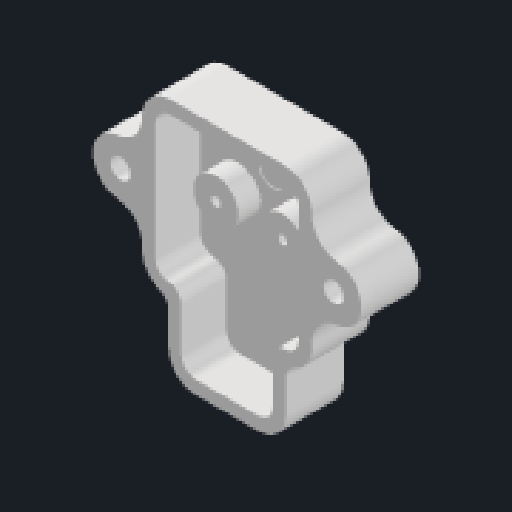
# Autodesk Inventor part: pressure_housing
Saved by Autodesk Inventor 2024 (Build 280153000, 153)
## iProperties
Created: 2025-03-06
Part Number: pressure_housing
Material: Generic
Document SubType Name: Modeling
Designer: colel
Density: 1 g/cm^3
Appearance: Default
Author: colel
Autodesk Inventor part; units mm, degrees
ref_plane "YZ Plane" through (0, 0, 0) normal (1, 0, 0) x (0, 1, 0)
ref_plane "XZ Plane" through (0, 0, 0) normal (0, 1, 0) x (-1, 0, 0)
ref_plane "XY Plane" through (0, 0, 0) normal (0, 0, 1) x (1, 0, 0)
sketch "Sketch1" plane through (0, 0, 0) normal (0, 0, 1) x (1, 0, 0)
  circle A0 centre (0, 0) radius 3
  circle A1 centre (7.5, -7) radius 1
  circle A2 centre (-7.5, -7) radius 1
  line L0 (-7.5, -7) -> (7.5, -7) construction
  line L1 (-19.05, 12.7) -> (19.05, 12.7)
  line L2 (19.05, 12.7) -> (19.05, -26.05)
  line L3 (19.05, -26.05) -> (-19.05, -26.05)
  line L4 (-19.05, -26.05) -> (-19.05, 12.7)
  circle A3 centre (-7.5, -7) radius 5
  circle A4 centre (7.5, -7) radius 5
  line L5 (16.05, 9.7) -> (-16.05, 9.7)
  line L6 (-16.05, 9.7) -> (-16.05, -23.05)
  line L7 (-16.05, -23.05) -> (16.05, -23.05)
  line L8 (16.05, -23.05) -> (16.05, 9.7)
  point P0 (0, -7)
  point P1 (0, 12.7)
  point P2 (16.05, -10.1819)
  point P3 (16.05, -2.5181)
  point P4 (-16.05, -2.5181)
  point P5 (-16.05, -10.1819)
  dimension "d0" = 7
  dimension "d1" = 15
  dimension "d2" = 6
  dimension "d3" = 2
  dimension "d4" = 38.1
  dimension "d5" = 12.7
  dimension "d6" = 19.05
  dimension "d7" = 4
  dimension "d8" = 3
  constraints: 18 end point, 5 centre point, 4 parallel, 3 coincident, 2 equal radius, 2 horizontal, 2 midpoint, 2 perpendicular, 2 vertical alignment, 1 horizontal alignment, 3 other
  measures "d0" distance from line of point (0, 0) L0
  measures "d1" distance of L0.start L0.end
  measures "d2" diameter of A0
  measures "d3" diameter of A2
  measures "d4" distance of L1.start L1.end
  measures "d5" distance from line of L1 point (0, 0)
  measures "d6" distance between parallel lines of L3 L0
  measures "d7" radial gap between concentric circles of A3 A2
  measures "d8" distance between parallel lines of L1 L5
extrude "Extrusion1" add sketch "Sketch1" against normal blind 3 contours A0 | A1 | A2 | L1 L2 L3 L4 | A3 | A4 | L8 L7 L6 L5
extrude "Extrusion2" add sketch "Sketch1" along normal blind 10 contours L1 L2 L3 L4
extrude "Extrusion3" add sketch "Sketch1" along normal blind 5 contours A3 | A4
extrude "Extrusion4" cut sketch "Sketch1" against normal blind 0.25 contours A0
fillet "Fillet1" radius 3.175 4 edges at (16.05, 9.7, 5) (16.05, -23.05, 5) (-16.05, -23.05, 5) (-16.05, 9.7, 5)
fillet "Fillet2" radius 6.175 4 edges at (-19.05, 12.7, 3.5) (-19.05, -26.05, 3.5) (19.05, -26.05, 3.5) (19.05, 12.7, 3.5)
sketch "Sketch2" plane through (0, 0, -3) normal (0, 0, -1) x (-1, 0, 0)
  line L0 (-7.075, -32.6439) -> (5.625, -32.6439) projected
  arc A0 (5.625, -38.9939) -> (5.625, -32.6439) centre (5.625, -35.8189) ccw projected
  line L1 (5.625, -38.9939) -> (-7.075, -38.9939) projected
  arc A1 (-7.075, -32.6439) -> (-7.075, -38.9939) centre (-7.075, -35.8189) ccw projected
  circle A2 centre (-22.0588, 28.4811) radius 1.5 projected
  circle A3 centre (32.925, -38.8189) radius 1.5 projected
  circle A4 centre (32.925, 7.1488) radius 1.5 projected
  circle A5 centre (-34.375, 7.1488) radius 1.5 projected
  circle A6 centre (-34.375, -38.8189) radius 1.5 projected
  circle A7 centre (20.6088, 28.4811) radius 1.5 projected
  arc A8 (39.275, 7.1488) -> (38.4243, 10.3238) centre (32.925, 7.1488) ccw projected
  line L2 (26.1081, 31.6561) -> (38.4243, 10.3238) projected
  arc A9 (26.1081, 31.6561) -> (20.6088, 34.8311) centre (20.6088, 28.4811) ccw projected
  line L3 (20.6088, 34.8311) -> (-22.0588, 34.8311) projected
  arc A10 (-22.0588, 34.8311) -> (-27.5581, 31.6561) centre (-22.0588, 28.4811) ccw projected
  line L4 (-39.8743, 10.3238) -> (-27.5581, 31.6561) projected
  arc A11 (-39.8743, 10.3238) -> (-40.725, 7.1488) centre (-34.375, 7.1488) ccw projected
  line L5 (-40.725, -38.8189) -> (-40.725, 7.1488) projected
  arc A12 (-40.725, -38.8189) -> (-34.375, -45.1689) centre (-34.375, -38.8189) ccw projected
  line L6 (32.925, -45.1689) -> (-34.375, -45.1689) projected
  arc A13 (32.925, -45.1689) -> (39.275, -38.8189) centre (32.925, -38.8189) ccw projected
  line L7 (39.275, 7.1488) -> (39.275, -38.8189) projected
  circle A14 centre (0, 0) radius 3 projected
  arc A15 (-12.875, 12.7) -> (-19.05, 6.525) centre (-12.875, 6.525) ccw projected
  line L8 (-19.05, 6.525) -> (-19.05, -19.875) projected
  arc A16 (-19.05, -19.875) -> (-12.875, -26.05) centre (-12.875, -19.875) ccw projected
  line L9 (-12.875, -26.05) -> (12.875, -26.05) projected
  arc A17 (12.875, -26.05) -> (19.05, -19.875) centre (12.875, -19.875) ccw projected
  line L10 (19.05, -19.875) -> (19.05, 6.525) projected
  arc A18 (19.05, 6.525) -> (12.875, 12.7) centre (12.875, 6.525) ccw projected
  line L11 (12.875, 12.7) -> (-12.875, 12.7) projected
  line L12 (-13.25, -45.1689) -> (-13.25, -26.0386)
  line L13 (-12.875, -26.05) -> (12.875, -26.05) projected
  line L14 (13.25, -45.1689) -> (13.25, -26.0386)
  line L15 (-13.25, -35.8189) -> (13.25, -35.8189) construction
  line L16 (-7.075, -41.9939) -> (7.075, -41.9939)
  arc A19 (5.625, -41.9939) -> (5.625, -29.6439) centre (5.625, -35.8189) ccw construction
  line L17 (7.075, -29.6439) -> (-7.075, -29.6439)
  arc A20 (-7.075, -29.6439) -> (-7.075, -41.9939) centre (-7.075, -35.8189) ccw
  arc A21 (6.35, -29.6866) -> (6.35, -41.9512) centre (7.075, -35.8189) ccw construction
  arc A22 (7.075, -41.9939) -> (7.075, -29.6439) centre (7.075, -35.8189) ccw
  line L18 (12.875, -26.05) -> (-12.875, -26.05) projected
  line L19 (-10.25, -26.05) -> (-10.25, -30.5227)
  line L20 (10.25, -26.05) -> (10.25, -30.5227)
  line L21 (-10.25, -30.5227) -> (-10.25, -35.8189)
  line L22 (10.25, -30.5227) -> (10.25, -35.8189)
  circle A23 centre (7.075, -35.8189) radius 3.175
  line L23 (5.625, -38.9939) -> (7.075, -38.9939)
  circle A24 centre (23.9875, -6.35) radius 1.5 projected
  circle A25 centre (-23.9875, -6.35) radius 1.5 projected
  point P0 (0, 0)
  point P1 (0, -35.8189)
  point P2 (0, -26.05)
  point P3 (-13.25, -35.8189)
  dimension "d19" = 6.175
  dimension "d20" = 3
  dimension "d21" = 3
  constraints: 20 end point, 17 point on circle, 11 point on line, 5 centre point, 3 perpendicular, 3 tangent, 2 midpoint, 2 vertical, 1 coincident, 1 parallel, 1 vertical alignment
  measures "d19" distance from line of L12 A1.centre
  measures "d20" distance between parallel lines of L19 L12
  measures "d21" distance between parallel lines of L14 L20
extrude "Extrusion5" add sketch "Sketch2" against normal up to surface (13 mm away) contours A1 L1 L23 A23 L22 A22 L16 A20 L21 | A20 L12 A16 L9 L19 | L20 L9 A17 L14 A22
sketch "Sketch3" plane through (0, 0, -3) normal (0, 0, -1) x (-1, 0, 0)
  line L0 (-10.25, -26.05) -> (10.25, -26.05) projected
  line L1 (10.25, -26.05) -> (10.25, -35.8189) projected
  arc A0 (7.075, -38.9939) -> (10.25, -35.8189) centre (7.075, -35.8189) ccw projected
  line L2 (7.075, -38.9939) -> (-7.075, -38.9939) projected
  arc A1 (-10.25, -35.8189) -> (-7.075, -38.9939) centre (-7.075, -35.8189) ccw projected
  line L3 (-10.25, -35.8189) -> (-10.25, -26.05) projected
  line L4 (-13.25, -26.0386) -> (-13.25, -35.8189) projected
  arc A2 (-13.25, -35.8189) -> (-7.075, -41.9939) centre (-7.075, -35.8189) ccw projected
  line L5 (-7.075, -41.9939) -> (7.075, -41.9939) projected
  arc A3 (7.075, -41.9939) -> (13.25, -35.8189) centre (7.075, -35.8189) ccw projected
  line L6 (13.25, -35.8189) -> (13.25, -26.0386) projected
  arc A4 (13.25, -26.0386) -> (19.05, -19.875) centre (12.875, -19.875) ccw projected
  line L7 (19.05, -19.875) -> (19.05, 6.525) projected
  arc A5 (19.05, 6.525) -> (12.875, 12.7) centre (12.875, 6.525) ccw projected
  line L8 (12.875, 12.7) -> (-12.875, 12.7) projected
  arc A6 (-12.875, 12.7) -> (-19.05, 6.525) centre (-12.875, 6.525) ccw projected
  line L9 (-19.05, 6.525) -> (-19.05, -19.875) projected
  arc A7 (-19.05, -19.875) -> (-13.25, -26.0386) centre (-12.875, -19.875) ccw projected
  point P0 (0, 0)
extrude "Extrusion6" add sketch "Sketch3" against normal blind 3 contours L0 L1 A0 L2 A1 L3
sketch "Sketch4" plane through (0, 0, 10) normal (0, 0, 1) x (1, 0, 0)
  arc A0 (13.25, -26.0386) -> (19.05, -19.875) centre (12.875, -19.875) ccw projected
  line L0 (19.05, -19.875) -> (19.05, 6.525) projected
  arc A1 (19.05, 6.525) -> (12.875, 12.7) centre (12.875, 6.525) ccw projected
  line L1 (12.875, 12.7) -> (-12.875, 12.7) projected
  arc A2 (-12.875, 12.7) -> (-19.05, 6.525) centre (-12.875, 6.525) ccw projected
  line L2 (-19.05, 6.525) -> (-19.05, -19.875) projected
  arc A3 (-19.05, -19.875) -> (-13.25, -26.0386) centre (-12.875, -19.875) ccw projected
  line L3 (-13.25, -35.8189) -> (-13.25, -26.0386) projected
  arc A4 (-13.25, -35.8189) -> (-7.075, -41.9939) centre (-7.075, -35.8189) ccw projected
  line L4 (7.075, -41.9939) -> (-7.075, -41.9939) projected
  arc A5 (7.075, -41.9939) -> (13.25, -35.8189) centre (7.075, -35.8189) ccw projected
  line L5 (13.25, -26.0386) -> (13.25, -35.8189) projected
  line L6 (10.25, -35.8189) -> (10.25, -26.05) projected
  arc A6 (7.075, -38.9939) -> (10.25, -35.8189) centre (7.075, -35.8189) ccw projected
  line L7 (-7.075, -38.9939) -> (7.075, -38.9939) projected
  arc A7 (-10.25, -35.8189) -> (-7.075, -38.9939) centre (-7.075, -35.8189) ccw projected
  line L8 (-10.25, -26.05) -> (-10.25, -35.8189) projected
  line L9 (-10.25, -26.05) -> (10.25, -26.05) projected
  line L10 (-12.875, 9.7) -> (12.875, 9.7) projected
  arc A8 (16.05, 6.525) -> (12.875, 9.7) centre (12.875, 6.525) ccw projected
  line L11 (16.05, 6.525) -> (16.05, -19.875) projected
  arc A9 (12.875, -23.05) -> (16.05, -19.875) centre (12.875, -19.875) ccw projected
  line L12 (12.875, -23.05) -> (-12.875, -23.05) projected
  arc A10 (-16.05, -19.875) -> (-12.875, -23.05) centre (-12.875, -19.875) ccw projected
  line L13 (-16.05, -19.875) -> (-16.05, 6.525) projected
  arc A11 (-12.875, 9.7) -> (-16.05, 6.525) centre (-12.875, 6.525) ccw projected
  line L14 (-10.25, -26.05) -> (-10.25, -23.05)
  line L15 (10.25, -26.05) -> (10.25, -23.05)
  point P0 (0, 0)
  constraints: 4 end point, 2 point on line, 2 vertical
extrude "Extrusion7" cut sketch "Sketch4" against normal up to surface (10 mm away) contours L9 L14 L12 L15
fillet "Fillet3" radius 3 4 edges at (-10.25, -23.05, 5) (-13.25, -26.0386, 3.5) (13.25, -26.0386, 3.5) (10.25, -23.05, 5)
sketch "Sketch5" plane through (0, 0, -3) normal (0, 0, -1) x (-1, 0, 0)
  arc A0 (-10.25, -26.0386) -> (-13.0678, -23.0441) centre (-13.25, -26.0386) ccw projected
  line L0 (-10.25, -35.8189) -> (-10.25, -26.0386) projected
  arc A1 (-10.25, -35.8189) -> (-7.075, -38.9939) centre (-7.075, -35.8189) ccw projected
  line L1 (7.075, -38.9939) -> (-7.075, -38.9939) projected
  arc A2 (7.075, -38.9939) -> (10.25, -35.8189) centre (7.075, -35.8189) ccw projected
  line L2 (10.25, -35.8189) -> (10.25, -26.0386) projected
  arc A3 (13.0678, -23.0441) -> (10.25, -26.0386) centre (13.25, -26.0386) ccw projected
  arc A4 (13.0678, -23.0441) -> (16.05, -19.875) centre (12.875, -19.875) ccw projected
  line L3 (16.05, -19.875) -> (16.05, 6.525) projected
  arc A5 (16.05, 6.525) -> (12.875, 9.7) centre (12.875, 6.525) ccw projected
  line L4 (12.875, 9.7) -> (-12.875, 9.7) projected
  arc A6 (-12.875, 9.7) -> (-16.05, 6.525) centre (-12.875, 6.525) ccw projected
  line L5 (-16.05, 6.525) -> (-16.05, -19.875) projected
  arc A7 (-16.05, -19.875) -> (-13.0678, -23.0441) centre (-12.875, -19.875) ccw projected
  arc A8 (-19.05, -19.875) -> (-15.1465, -25.617) centre (-12.875, -19.875) ccw projected
  line L6 (-19.05, -19.875) -> (-19.05, 6.525) projected
  arc A9 (-12.875, 12.7) -> (-19.05, 6.525) centre (-12.875, 6.525) ccw projected
  line L7 (-12.875, 12.7) -> (12.875, 12.7) projected
  arc A10 (19.05, 6.525) -> (12.875, 12.7) centre (12.875, 6.525) ccw projected
  line L8 (19.05, 6.525) -> (19.05, -19.875) projected
  arc A11 (15.1465, -25.617) -> (19.05, -19.875) centre (12.875, -19.875) ccw projected
  arc A12 (15.1465, -25.617) -> (13.25, -28.4067) centre (16.25, -28.4067) ccw projected
  line L9 (13.25, -35.8189) -> (13.25, -28.4067) projected
  arc A13 (7.075, -41.9939) -> (13.25, -35.8189) centre (7.075, -35.8189) ccw projected
  line L10 (-7.075, -41.9939) -> (7.075, -41.9939) projected
  arc A14 (-13.25, -35.8189) -> (-7.075, -41.9939) centre (-7.075, -35.8189) ccw projected
  line L11 (-13.25, -28.4067) -> (-13.25, -35.8189) projected
  arc A15 (-13.25, -28.4067) -> (-15.1465, -25.617) centre (-16.25, -28.4067) ccw projected
  line L12 (16.05, -19.875) -> (16.05, 6.525) projected
  line L13 (-16.05, 6.525) -> (-16.05, -19.875) projected
  line L14 (-16.05, -6.675) -> (-19.05, -6.675) construction
  line L15 (16.05, -6.675) -> (19.05, -6.675) construction
  line L16 (17.55, -3.591) -> (17.55, -9.759) construction
  line L17 (-17.55, -3.591) -> (-17.55, -9.759) construction
  arc A16 (-19.05, -2.5181) -> (-19.05, -10.1819) centre (-23.9875, -6.35) ccw
  circle A17 centre (-23.9875, -6.35) radius 2.25
  arc A18 (19.05, -10.1819) -> (19.05, -2.5181) centre (23.9875, -6.35) ccw
  circle A19 centre (23.9875, -6.35) radius 2.25
  arc A20 (16.05, 6.525) -> (12.875, 9.7) centre (12.875, 6.525) ccw projected
  line L18 (16.05, -19.875) -> (16.05, 6.525) projected
  arc A21 (13.0678, -23.0441) -> (16.05, -19.875) centre (12.875, -19.875) ccw projected
  arc A22 (13.0678, -23.0441) -> (10.25, -26.0386) centre (13.25, -26.0386) ccw projected
  line L19 (10.25, -26.0386) -> (10.25, -23.05) projected
  line L20 (-10.25, -23.05) -> (10.25, -23.05) projected
  line L21 (-10.25, -23.05) -> (-10.25, -26.0386) projected
  arc A23 (-10.25, -26.0386) -> (-13.0678, -23.0441) centre (-13.25, -26.0386) ccw projected
  arc A24 (-16.05, -19.875) -> (-13.0678, -23.0441) centre (-12.875, -19.875) ccw projected
  arc A25 (-12.875, 9.7) -> (-16.05, 6.525) centre (-12.875, 6.525) ccw projected
  line L22 (12.875, 9.7) -> (-12.875, 9.7) projected
  arc A26 (16.05, 6.525) -> (12.875, 9.7) centre (12.875, 6.525) ccw projected
  arc A27 (13.0678, -23.0441) -> (16.05, -19.875) centre (12.875, -19.875) ccw projected
  arc A28 (13.0678, -23.0441) -> (10.25, -26.0386) centre (13.25, -26.0386) ccw projected
  line L23 (10.25, -26.0386) -> (10.25, -23.05) projected
  line L24 (-10.25, -23.05) -> (10.25, -23.05) projected
  line L25 (-10.25, -23.05) -> (-10.25, -26.0386) projected
  arc A29 (-10.25, -26.0386) -> (-13.0678, -23.0441) centre (-13.25, -26.0386) ccw projected
  arc A30 (-16.05, -19.875) -> (-13.0678, -23.0441) centre (-12.875, -19.875) ccw projected
  line L26 (-16.05, 6.525) -> (-16.05, -19.875) projected
  arc A31 (-12.875, 9.7) -> (-16.05, 6.525) centre (-12.875, 6.525) ccw projected
  line L27 (12.875, 9.7) -> (-12.875, 9.7) projected
  point P0 (0, 0)
  point P1 (-17.55, -6.675)
  point P2 (17.55, -6.675)
  point P3 (-19.05, -2.5181)
  point P4 (-19.05, -10.1819)
  point P5 (19.05, -10.1819)
  point P6 (19.05, -2.5181)
  constraints: 8 end point, 8 midpoint, 4 centre point, 4 point on circle, 2 vertical
extrude "Extrusion8" add sketch "Sketch5" against normal blind 3 contours A17 | A19
extrude "Extrusion9" add sketch "Sketch5" against normal up to surface (13 mm away) contours A16 L6 | A18 L8
fillet "Fillet4" radius 6.35 4 edges at (19.05, -2.5181, 3.5) (19.05, -10.1819, 3.5) (-19.05, -2.5181, 3.5) (-19.05, -10.1819, 3.5)
body "Solid1"
